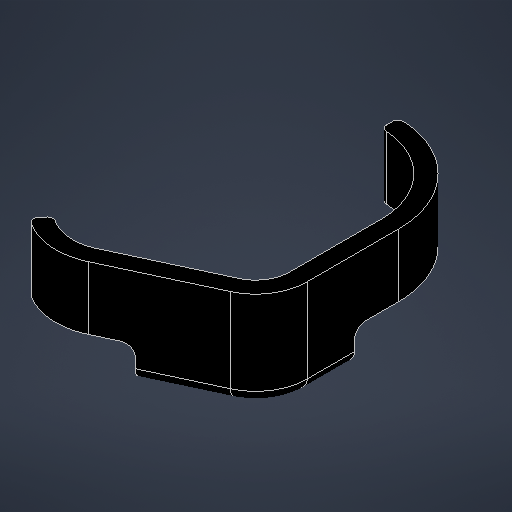
# Autodesk Inventor part: Dribbler Cover
Saved by Autodesk Inventor 2026.1 (Build 301233020, 233B)
## iProperties
Created: 2026-04-16
Part Number: Dribbler Cover
Material: Generic
Document SubType Name: Modeling
Designer: Bahaa
Mass: 3.1542 g
Surface Area: 27.6407 cm^2
Volume: 3.1542 cm^3
Density: 1 g/cm^3
Appearance: Default(1)
Author: Bahaa
Autodesk Inventor part; units mm, degrees
ref_plane "YZ Plane" through (0, 0, 0) normal (1, 0, 0) x (0, 1, 0)
ref_plane "XZ Plane" through (0, 0, 0) normal (0, 1, 0) x (-1, 0, 0)
ref_plane "Work Plane1" through (0, 0, 0) normal (0, 0, 1) x (1, 0, 0)
sketch "Sketch1" plane through (0, 0, 0) normal (0, 0, 1) x (1, 0, 0)
  arc A0 (14.9, 13.3274) -> (-10.4833, 15.6726) centre (2.1, 13.3274) ccw
  line L0 (14.9, -2.5791) -> (14.9, 13.3274)
  arc A1 (12.0131, -7.1106) -> (14.9, -2.5791) centre (9.9, -2.5791) ccw
  line L1 (-4.9417, -15.0167) -> (12.0131, -7.1106)
  arc A2 (-14.7815, -7.3901) -> (-4.9417, -15.0167) centre (-7.9, -8.6726) ccw
  arc A3 (15.9, 13.3274) -> (2.1, 27.1274) centre (2.1, 13.3274) ccw
  line L2 (15.9, 13.3274) -> (15.9, -2.5791)
  arc A4 (12.4357, -8.0169) -> (15.9, -2.5791) centre (9.9, -2.5791) ccw
  line L3 (12.4357, -8.0169) -> (-4.5191, -15.923)
  arc A5 (-13.0423, -14.8009) -> (-4.5191, -15.923) centre (-7.9, -8.6726) ccw
  arc A6 (-14.9707, -17.0991) -> (-3.2512, -18.642) centre (-7.9, -8.6726) ccw
  line L4 (-3.2512, -18.642) -> (13.7036, -10.7358)
  arc A7 (13.7036, -10.7358) -> (18.9, -2.5791) centre (9.9, -2.5791) ccw
  line L5 (18.9, -2.5791) -> (18.9, 13.3274)
  arc A8 (18.9, 13.3274) -> (2.1, 30.1274) centre (2.1, 13.3274) ccw
  line L6 (2.1, 13.3274) -> (2.1, 30.1274)
  line L7 (-7.9, -8.6726) -> (-14.9707, -17.0991)
  line L8 (-7.9, -8.6726) -> (3.1, -8.6726) construction
  circle A9 centre (11.641, 2.6757) radius 3
  circle A10 centre (2.1, -8.423) radius 3
  line L9 (11.641, -0.3243) -> (18.9, -0.3243)
  line L10 (11.641, 5.6757) -> (18.9, 5.6757)
  line L11 (7.7773, -13.4993) -> (4.8189, -7.1552)
  line L12 (-0.6189, -9.6909) -> (2.3394, -16.035)
  arc A11 (13.9, 13.3274) -> (-9.5003, 15.4894) centre (2.1, 13.3274) ccw
  line L13 (13.9, 13.3274) -> (13.9, -2.5791)
  arc A12 (11.5905, -6.2043) -> (13.9, -2.5791) centre (9.9, -2.5791) ccw
  line L14 (11.5905, -6.2043) -> (-5.3643, -14.1104)
  arc A13 (-13.7984, -7.5733) -> (-5.3643, -14.1104) centre (-7.9, -8.6726) ccw
  point P0 (0, 0)
  point P1 (15.9, -0.3243)
  point P2 (15.9, 5.6757)
  point P3 (6.5094, -10.7804)
  point P4 (1.0715, -13.3161)
  point P5 (-11.7567, -13.2688)
  point P6 (0.2263, -11.5035)
  point P7 (13.9, 5.6757)
  point P8 (2.1, 25.1274)
  point P9 (13.9, -0.3243)
  point P10 (5.6642, -8.9678)
  point P11 (6.0868, -9.8741)
  point P12 (14.9, -0.3243)
  point P13 (14.9, 5.6757)
  point P14 (2.1, 26.1274)
  point P15 (0.6489, -12.4098)
  point P16 (-12.3995, -14.0349)
extrude "Extrusion1" add sketch "Sketch1" along normal blind 8 and the other way blind 6.7 contours L6 A8 L5 L10 L2 A3 | L10 L5 L9 L2 | L9 L5 A7 L4 L11 L3 A4 L2 | L11 L4 L12 L3 | L12 L4 A6 L7 A5 L3
extrude "Extrusion2" add sketch "Sketch1" against normal blind 2 from surface at -6.7 contours A0 L6 A3 L2 L10 L0 | L10 L2 L9 L0 | L0 L9 L13 A9 L10 | L6 A8 L5 L10 L2 A3 | L9 L2 A4 L3 L11 L1 A1 L0 | L13 A9 L10 | L10 L5 L9 L2 | L9 A9 L13 | L9 L5 A7 L4 L11 L3 A4 L2 | A9 L13 | A9 L13 | L11 L3 L12 L1 | L1 A10 L14 L11 | L1 L12 L14 A10 | A10 L14 | L11 L4 L12 L3 | L14 A10 L11 | L12 L3 A5 L7 A2 L1 | L14 L12 A10 | A10 L14 | L12 L4 A6 L7 A5 L3
extrude "Extrusion3" cut sketch "Sketch1" along normal blind 5.7 from surface at -8.7 contours A0 L6 A3 L2 L10 L0 | L6 A8 L5 L10 L2 A3 | L9 L2 A4 L3 L11 L1 A1 L0 | L12 L3 A5 L7 A2 L1 | L12 L4 A6 L7 A5 L3
sketch "Sketch2" plane through (18.9, -2.5791, -8.7) normal (0, 0, -1) x (-1, 0, 0)
  arc A0 (7.259, 2.2548) -> (7.259, 8.2548) centre (7.259, 5.2548) ccw projected
  arc A1 (19.5189, -7.1118) -> (14.0811, -4.5761) centre (16.8, -5.844) ccw projected
  point P0 (18.9, 2.5791)
  point P1 (6.5605, 2.2699)
  point P2 (18.5189, -7.1118)
  point P3 (13.0811, -4.5761)
  point P4 (6.7036, 2.2879)
  point P5 (6.7036, 8.2216)
hole "Hole1" at (11.641, 2.6757, -8.7) at (2.1, -8.423, -8.7) direction (0, 0, 1) diameter 2.9 end through all countersink diameter 5.5 countersink angle 90 clearance for "Countersunk Flat Head Screw ISO 2009/7046" size "M2.5" standard "ISO"
fillet "Fillet2" radius 1 6 edges at (2.1, 27.1274, 2.5) (2.1, 30.1274, 2.5) (-13.0423, -14.8009, 2.5) (-14.9707, -17.0991, 2.5) (3.7905, -12.0482, -6.7) (15.9, 2.6757, -6.7)
fillet "Fillet3" radius 2 5 edges at (1.7055, -14.6756, -3) (17.4905, -7.4148, -8.7) (8.0215, -13.3854, -8.7) (18.9, 1.5483, -8.7) (17.4, 5.6757, -3)
equation "\"d4\" = d1"
equation "\"d5\" = d1"
equation "\"d6\" = d1 + d7 + d0"
equation "\"d8\" = d1 + d9 + d0"
equation "\"d1\" = 3"
equation "\"d7\" = 7"
equation "\"d0\" = 1"
equation "\"d9\" = 12.8"
body "Solid1"
